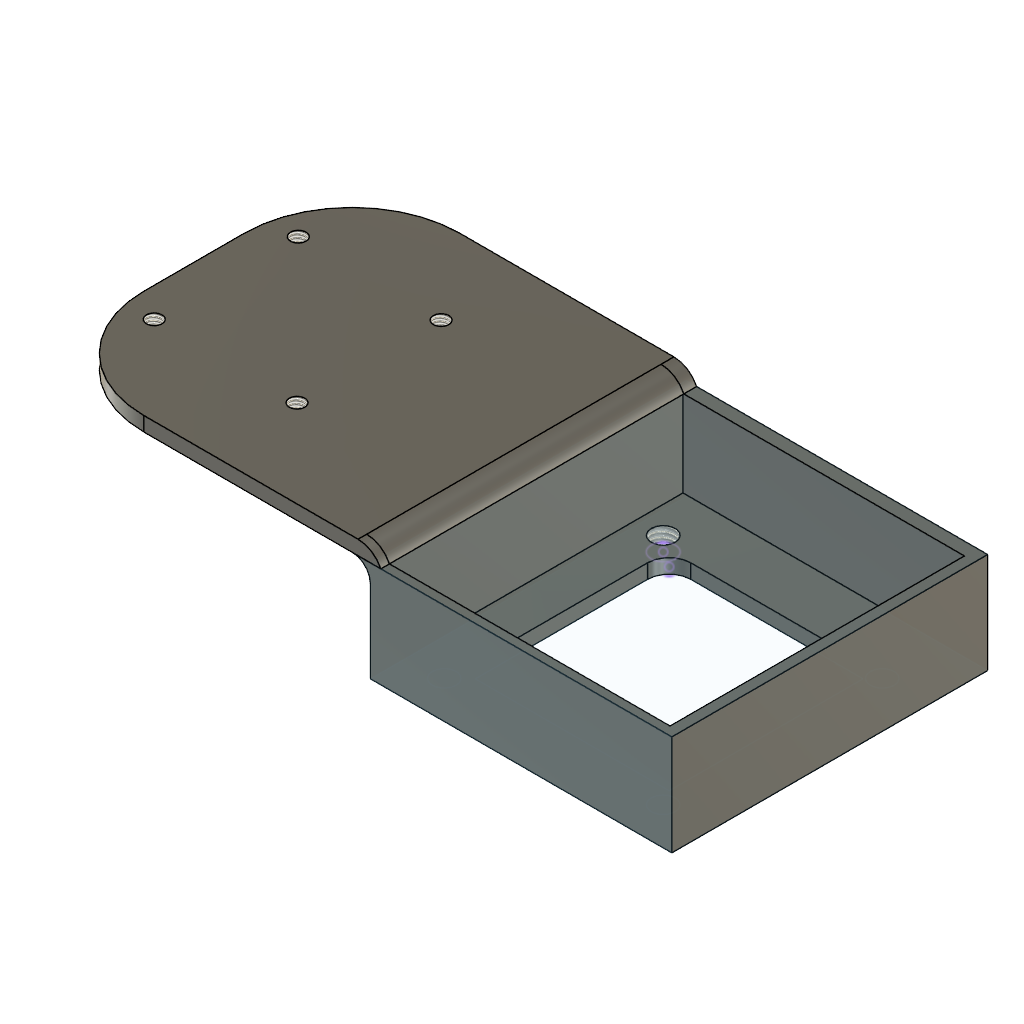
container (Autodesk Fusion 360 design; units mm, degrees)
part number: 2026-09-24-19-30-31-447
Autodesk Fusion 360 part; units mm, degrees
sketch "Sketch1" plane through (0, 0, 0) normal (0, 0, 1) x (1, 0, 0)
  line L0 (2.4087, -20.2064) -> (44.4087, -20.2064)
  line L1 (44.4087, -20.2064) -> (44.4087, 23.7936)
  line L2 (44.4087, 23.7936) -> (2.4087, 23.7936)
  line L3 (2.4087, 23.7936) -> (2.4087, -20.2064)
  dimension "d1" = 42
  dimension "d2" = 44
  constraint horizontal L0
  constraint vertical L1
  constraint horizontal L2
  constraint vertical L3
  measures "d1" distance of L0.start L0.end
  measures "d2" distance of L0.start L2.end
extrude "Extrude1" add sketch "Sketch1" along normal blind 14
sketch "Sketch2" plane through (0, 0, 14) normal (0, 0, 1) x (-1, 0, 0)
  line L0 (-2.4087, -23.7936) -> (-2.4087, 20.2064)
  line L1 (-2.4087, 20.2064) -> (-44.4087, 20.2064)
  line L2 (-44.4087, 20.2064) -> (-44.4087, -23.7936)
  line L3 (-44.4087, -23.7936) -> (-2.4087, -23.7936)
sketch "Sketch3" plane through (0, 0, 14) normal (0, 0, 1) x (-1, 0, 0)
sketch "Sketch4" plane through (0, 0, 14) normal (0, 0, 1) x (-1, 0, 0)
  line L0 (-3.7615, -21.9929) -> (-42.9615, -21.9929)
  line L1 (-42.9615, -21.9929) -> (-42.9615, 19.0071)
  line L2 (-42.9615, 19.0071) -> (-3.7615, 19.0071)
  line L3 (-3.7615, 19.0071) -> (-3.7615, -21.9929)
  dimension "d7" = 39.2
  dimension "d8" = 41
  constraint horizontal L0
  constraint vertical L1
  constraint horizontal L2
  constraint vertical L3
  measures "d7" distance of L0.start L0.end
  measures "d8" distance of L0.start L2.end
extrude "Extrude2" cut sketch "Sketch4" against normal blind 12
sketch "Sketch5" plane through (0, 0, 14) normal (0, 0, 1) x (-1, 0, 0)
  line L0 (-9.7202, -14.1091) -> (-36.7202, -14.1091)
  line L1 (-36.7202, -14.1091) -> (-36.7202, 12.8909)
  line L2 (-36.7202, 12.8909) -> (-9.7202, 12.8909)
  line L3 (-9.7202, 12.8909) -> (-9.7202, -14.1091)
  dimension "d11" = 27
  dimension "d12" = 27
  constraint horizontal L0
  constraint vertical L1
  constraint horizontal L2
  constraint vertical L3
  measures "d11" distance of L0.start L0.end
  measures "d12" distance of L0.start L2.end
extrude "Extrude3" cut sketch "Sketch5" against normal blind 16
sketch "Sketch6" plane through (0, 0, 0) normal (0, 0, -1) x (1, 0, 0)
  line L0 (2.4087, 20.2064) -> (2.4087, -23.7936)
  line L1 (2.4087, -23.7936) -> (44.4087, -23.7936)
  line L2 (44.4087, -23.7936) -> (44.4087, 20.2064)
  line L3 (44.4087, 20.2064) -> (2.4087, 20.2064)
  circle A0 centre (7.5, 15) radius 1.6
  circle A1 centre (38, 15) radius 1.6
  circle A2 centre (7.5041, -15.5) radius 1.6
  circle A3 centre (38.0041, -15.5) radius 1.6
  line L4 (36.7202, 12.8909) -> (36.7202, -14.1091)
  line L5 (36.7202, -14.1091) -> (9.7202, -14.1091)
  line L6 (9.7202, -14.1091) -> (9.7202, 12.8909)
  line L7 (9.7202, 12.8909) -> (36.7202, 12.8909)
  dimension "d15" = 3.2
  dimension "d16" = 3.2
  dimension "d17" = 3.2
  dimension "d18" = 3.2
  dimension "d19" = 30.5
  dimension "d20" = 30.5
  dimension "d21" = 30.5
  dimension "d22" = 30.5
  measures "d15" diameter of A0
  measures "d16" diameter of A1
  measures "d17" diameter of A2
  measures "d18" diameter of A3
  measures "d19" distance of A0.centre A1.centre
  measures "d20" vertical distance of A0.centre A2.centre
  measures "d21" distance of A2.centre A3.centre
  measures "d22" vertical distance of A1.centre A3.centre
extrude "Extrude4" cut sketch "Sketch6" against normal blind 8 contours A0 | A1 | A2 | A3
thread "Thread1" "ISO Metric profile 4.0 M4x0.7 M4x0.7 6H" major diameter 4.1095 minor diameter 3.332 pitch 0.7 angle 60 resizes the face on face at (9.0961, 15.6593, 0.6667)
thread "Thread2" "ISO Metric profile 4.0 M4x0.7 M4x0.7 6H" major diameter 4.1095 minor diameter 3.332 pitch 0.7 angle 60 resizes the face on face at (39.598, -14.9202, 1.3333)
thread "Thread3" "ISO Metric profile 4.0 M4x0.7 M4x0.7 6H" major diameter 4.1095 minor diameter 3.332 pitch 0.7 angle 60 resizes the face on face at (39.6021, 15.5798, 1.3333)
sketch "Sketch7" plane through (0, 0, 14) normal (0, 0, 1) x (-1, 0, 0)
  line L0 (-3.8753, 20.2126) -> (44.1247, 20.2126)
  line L1 (44.1247, 20.2126) -> (44.1247, -23.7874)
  line L2 (44.1247, -23.7874) -> (-3.8753, -23.7874)
  line L3 (-3.8753, -23.7874) -> (-3.8753, 20.2126)
  dimension "d31" = 48
  dimension "d32" = 44
  constraint horizontal L0
  constraint vertical L1
  constraint horizontal L2
  constraint vertical L3
  measures "d31" distance of L0.start L0.end
  measures "d32" distance of L0.start L2.end
extrude "Extrude5" add sketch "Sketch7" along normal blind 2
sketch "Sketch8" plane through (0, 0, 16) normal (0, 0, 1) x (-1, 0, 0)
  line L0 (-3.8753, -23.7874) -> (44.1247, -23.7874)
  line L1 (44.1247, -23.7874) -> (44.1247, 20.2126)
  line L2 (44.1247, 20.2126) -> (-3.8753, 20.2126)
  line L3 (-3.8753, 20.2126) -> (-3.8753, -23.7874)
  circle A0 centre (40, 7.8846) radius 1.1
  circle A1 centre (20, 8) radius 1.1
  circle A2 centre (19.9373, -11.9999) radius 1.1
  circle A3 centre (39.937, -12.1153) radius 1.1
  dimension "d35" = 2.2
  dimension "d36" = 2.2
  dimension "d37" = 2.2
  dimension "d38" = 2.2
  dimension "d39" = 20
  dimension "d40" = 20
  dimension "d41" = 20
  dimension "d42" = 20
  measures "d35" diameter of A0
  measures "d36" diameter of A1
  measures "d37" diameter of A2
  measures "d38" diameter of A3
  measures "d39" horizontal distance of A0.centre A1.centre
  measures "d40" distance of A0.centre A3.centre
  measures "d41" distance of A2.centre A3.centre
  measures "d42" distance of A1.centre A2.centre
extrude "Extrude6" cut sketch "Sketch8" against normal blind 4 contours A0 | A1 | A2 | A3
thread "Thread4" "ISO Metric profile 2.6 M2.6x0.45 M2.6x0.45 6H" major diameter 2.675 minor diameter 2.1754 pitch 0.45 angle 60 resizes the face on face at (-20.966, -8.5261, 15.3333)
thread "Thread5" "ISO Metric profile 2.6 M2.6x0.45 M2.6x0.45 6H" major diameter 2.675 minor diameter 2.1754 pitch 0.45 angle 60 resizes the face on face at (-41.0945, -7.7751, 15.3333)
thread "Thread6" "ISO Metric profile 2.6 M2.6x0.45 M2.6x0.45 6H" major diameter 2.675 minor diameter 2.1754 pitch 0.45 angle 60 resizes the face on face at (-18.9987, 12.5735, 14.6667)
thread "Thread7" "ISO Metric profile 2.6 M2.6x0.45 M2.6x0.45 6H" major diameter 2.675 minor diameter 2.1754 pitch 0.45 angle 60 resizes the face on face at (-38.9984, 12.6889, 14.6667)
thread "Thread8" "ISO Metric profile 4.0 M4x0.7 M4x0.7 6H" major diameter 4.1095 minor diameter 3.332 pitch 0.7 angle 60 resizes the face on face at (9.098, -14.9202, 1.3333)
sketch "Sketch9" plane through (44.4087, 0, 0) normal (1, 0, 0) x (0, 1, 0)
  line L0 (-20.2064, 0) -> (23.7936, 0)
  line L1 (23.7936, 0) -> (23.7936, 14)
  line L2 (23.7936, 14) -> (-20.2064, 14)
  line L3 (-20.2064, 14) -> (-20.2064, 0)
  circle A0 centre (0.7936, 7.9) radius 2.5
  dimension "d55" = 5
  dimension "d56" = 21
  dimension "d57" = 7.9
  measures "d55" diameter of A0
  measures "d56" distance of L3 A0.centre
  measures "d57" distance of L0 A0.centre
sketch "Sketch10" plane through (0, 0, 0) normal (0, 0, 1) x (1, 0, 0)
sketch "Sketch11" plane through (0, 0, 0) normal (0, 0, -1) x (1, 0, 0)
  line L0 (2.4087, 20.2064) -> (2.4087, -23.7936)
  line L1 (2.4087, -23.7936) -> (44.4087, -23.7936)
  line L2 (44.4087, -23.7936) -> (44.4087, 20.2064)
  line L3 (44.4087, 20.2064) -> (2.4087, 20.2064)
  line L4 (36.7202, 12.8909) -> (36.7202, -14.1091)
  line L5 (36.7202, -14.1091) -> (9.7202, -14.1091)
  line L6 (9.7202, -14.1091) -> (9.7202, 12.8909)
  line L7 (9.7202, 12.8909) -> (36.7202, 12.8909)
  circle A0 centre (7.5, 15) radius 1.666
  circle A1 centre (38, 15) radius 1.666
  circle A2 centre (38.0041, -15.5) radius 1.666
  circle A3 centre (7.5041, -15.5) radius 1.666
fillet "Fillet1" radius 2.5 1 edges at (2.4087, 1.7905, 14)
fillet "Fillet2" radius 3.5 1 edges at (3.8753, 1.7874, 16)
fillet "Fillet3" radius 3 1 edges at (36.7202, -12.8909, 1)
fillet "Fillet4" radius 3 1 edges at (9.7202, -12.8909, 1)
fillet "Fillet5" radius 3 1 edges at (9.7202, 14.1091, 1)
fillet "Fillet6" radius 3 1 edges at (36.7202, 14.1091, 1)
sketch "Sketch13" plane through (0, -20.2064, 0) normal (0, -1, 0) x (1, 0, 0)
  line L0 (2.4087, 0) -> (44.4087, 0)
  line L1 (44.4087, 0) -> (44.4087, 14)
  line L2 (44.4087, 14) -> (3.8753, 14)
  line L3 (3.8753, 14) -> (-0.0913, 14)
  arc A0 (2.4087, 11.5) -> (-0.0913, 14) centre (-0.0913, 11.5) ccw
  line L4 (2.4087, 11.5) -> (2.4087, 0)
fillet "Fillet7" radius 15 1 edges at (-44.1247, -20.2126, 15)
fillet "Fillet8" radius 15 1 edges at (-44.1247, 23.7874, 15)
